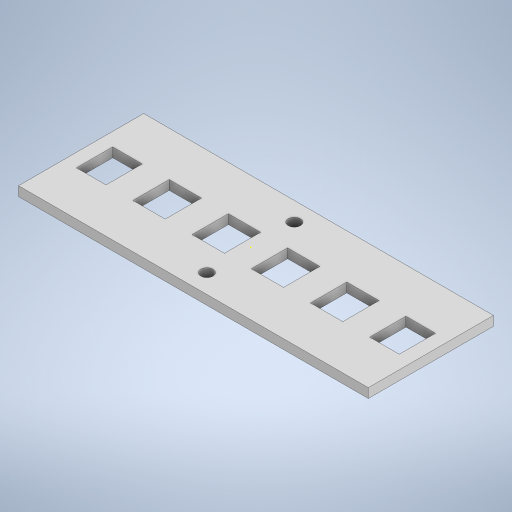
# Autodesk Inventor part: MILESTONE3LID
Saved by Autodesk Inventor 2024 (Build 280153000, 153)
## iProperties
Created: 2023-11-14
Part Number: MILESTONE3LID
Material: Generic
Document SubType Name: Modeling
Designer: Yuvraj
Density: 1 g/cm^3
Appearance: Default
Author: Yuvraj
Autodesk Inventor part; units mm, degrees
ref_plane "YZ Plane" through (0, 0, 0) normal (1, 0, 0) x (0, 1, 0)
ref_plane "XZ Plane" through (0, 0, 0) normal (0, 1, 0) x (-1, 0, 0)
ref_plane "XY Plane" through (0, 0, 0) normal (0, 0, 1) x (1, 0, 0)
sketch "Sketch1" plane through (0, 0, 0) normal (0, 1, 0) x (-1, 0, 0)
  line L0 (63, 23.25) -> (-67, 23.25)
  line L1 (-67, 23.25) -> (-67, -23.25)
  line L2 (-67, -23.25) -> (63, -23.25)
  line L3 (63, -23.25) -> (63, 23.25)
  point P0 (0, 0)
  dimension "d1" = 46.5
  dimension "d2" = 23.25
  dimension "d3" = 130
  dimension "d4" = 67
  constraints: 8 end point, 2 parallel, 1 horizontal, 1 perpendicular
  measures "d1" distance between parallel lines of L2 L0
  measures "d2" distance from line of point (0, 0) L0
  measures "d3" distance between parallel lines of L1 L3
  measures "d4" distance from line of point (0, 0) L1
extrude "Extrusion1" add sketch "Sketch1" along normal blind 3.5
sketch "Sketch3" plane through (0, 3.5, 0) normal (0, 1, 0) x (1, 0, 0)
  line L0 (-58, 6.75) -> (-47, 6.75)
  line L1 (-47, 6.75) -> (-47, -6.75)
  line L2 (-47, -6.75) -> (-58, -6.75)
  line L3 (-58, -6.75) -> (-58, 6.75)
  line L4 (-37, 6.75) -> (-25, 6.75)
  line L5 (-25, 6.75) -> (-25, -6.75)
  line L6 (-25, -6.75) -> (-37, -6.75)
  line L7 (-37, -6.75) -> (-37, 6.75)
  line L8 (-15, 6.75) -> (-3, 6.75)
  line L9 (-3, 6.75) -> (-3, -6.75)
  line L10 (-3, -6.75) -> (-15, -6.75)
  line L11 (-15, -6.75) -> (-15, 6.75)
  line L12 (7, 6.75) -> (19, 6.75)
  line L13 (19, 6.75) -> (19, -6.75)
  line L14 (19, -6.75) -> (7, -6.75)
  line L15 (7, -6.75) -> (7, 6.75)
  line L16 (29, 6.75) -> (41, 6.75)
  line L17 (41, 6.75) -> (41, -6.75)
  line L18 (41, -6.75) -> (29, -6.75)
  line L19 (29, -6.75) -> (29, 6.75)
  line L20 (51, 6.75) -> (62, 6.75)
  line L21 (62, 6.75) -> (62, -6.75)
  line L22 (62, -6.75) -> (51, -6.75)
  line L23 (51, -6.75) -> (51, 6.75)
  line L24 (67, 23.25) -> (-63, 23.25) projected
  line L25 (-63, -23.25) -> (67, -23.25) projected
  line L26 (-63, 23.25) -> (-63, -23.25) projected
  line L27 (67, -23.25) -> (67, 23.25) projected
  point P0 (0, 0)
  dimension "d21" = 16.5
  dimension "d22" = 16.5
  dimension "d23" = 5
  dimension "d24" = 10
  dimension "d25" = 10
  dimension "d26" = 10
  dimension "d27" = 10
  dimension "d28" = 5
  dimension "d29" = 16
  dimension "d30" = 38
  dimension "d31" = 60
  dimension "d32" = 60
  dimension "d33" = 38
  dimension "d34" = 16
  constraints: 48 end point, 12 parallel, 10 point on line, 6 horizontal, 6 perpendicular
  measures "d21" distance between parallel lines of L24 L0
  measures "d22" distance between parallel lines of L25 L18
  measures "d23" distance between parallel lines of L26 L3
  measures "d24" distance between parallel lines of L1 L7
  measures "d25" distance between parallel lines of L11 L5
  measures "d26" distance between parallel lines of L19 L13
  measures "d27" distance between parallel lines of L23 L17
  measures "d28" distance between parallel lines of L27 L21
  measures "d29" distance between parallel lines of L26 L1
  measures "d30" distance between parallel lines of L26 L5
  measures "d31" distance between parallel lines of L26 L9
  measures "d32" distance between parallel lines of L27 L15
  measures "d33" distance between parallel lines of L27 L19
  measures "d34" distance between parallel lines of L27 L23
extrude "Extrusion3" cut sketch "Sketch3" against normal blind 10 contours L0 L1 L2 L3 | L4 L5 L6 L7 | L8 L9 L10 L11 | L12 L13 L14 L15 | L16 L17 L18 L19 | L20 L21 L22 L23
sketch "Sketch4" plane through (0, 3.5, 0) normal (0, 1, 0) x (1, 0, 0)
  point P0 (0, 0)
sketch "Sketch5" plane through (0, 3.5, 0) normal (0, 1, 0) x (1, 0, 0)
  circle A0 centre (0, 16.25) radius 2.25
  circle A1 centre (0, -16.25) radius 2.25
  line L0 (67, 23.25) -> (-63, 23.25) projected
  line L1 (67, -23.25) -> (67, 23.25) projected
  line L2 (-63, -23.25) -> (67, -23.25) projected
  point P0 (0, 0)
  dimension "d37" = 4.5
  dimension "d38" = 4.5
  dimension "d39" = 7
  dimension "d40" = 67
  dimension "d41" = 7
  dimension "d42" = 67
  constraints: 2 centre point
  measures "d37" diameter of A1
  measures "d38" diameter of A0
  measures "d39" distance from line of L0 A0.centre
  measures "d40" distance from line of L1 A0.centre
  measures "d41" distance from line of L2 A1.centre
  measures "d42" distance from line of L1 A1.centre
extrude "Extrusion4" cut sketch "Sketch5" against normal blind 3.5
body "Solid1"
